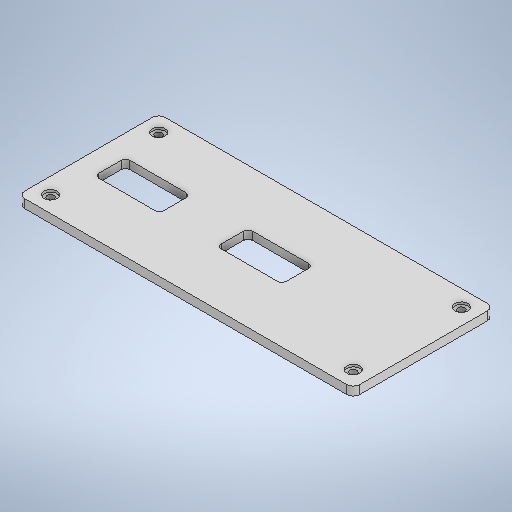
# Autodesk Inventor part: arcade_box_lid_iteration3
Saved by Autodesk Inventor 2025.2 (Build 292293000, 293)
## iProperties
Created: 2025-03-25
Part Number: arcade_box_lid_iteration3
Material: Generic
Document SubType Name: Modeling
Designer: osmon
Density: 1 g/cm^3
Appearance: Default
Author: osmon
Autodesk Inventor part; units mm, degrees
ref_plane "YZ Plane" through (0, 0, 0) normal (1, 0, 0) x (0, 1, 0)
ref_plane "XZ Plane" through (0, 0, 0) normal (0, 1, 0) x (-1, 0, 0)
ref_plane "XY Plane" through (0, 0, 0) normal (0, 0, 1) x (1, 0, 0)
sketch "Sketch1" plane through (0, 0, 0) normal (0, 1, 0) x (-1, 0, 0)
  line L0 (0, 0) -> (-155, 0)
  line L1 (-155, 0) -> (-155, -65)
  line L2 (-155, -65) -> (0, -65)
  line L3 (0, -65) -> (0, 0)
  dimension "d0" = 155
  dimension "d1" = 65
  constraints: 8 end point, 2 parallel, 1 horizontal, 1 perpendicular
  measures "d0" distance of L2.end L1.end
  measures "d1" distance of L1.end L0.end
extrude "Extrusion1" add sketch "Sketch1" along normal blind 4
sketch "Sketch2" plane through (0, 0, 0) normal (0, -1, 0) x (1, 0, 0)
  line L0 (155, 0) -> (155, -65) projected
  line L1 (0, 0) -> (155, 0) projected
  line L2 (0, -65) -> (0, 0) projected
  line L3 (155, -65) -> (0, -65) projected
  line L4 (3, -62) -> (3, -3)
  line L5 (3, -3) -> (152, -3)
  line L6 (152, -3) -> (152, -62)
  line L7 (152, -62) -> (3, -62)
  line L8 (152, -62) -> (143, -62)
  line L9 (143, -62) -> (143, -53)
  line L10 (143, -53) -> (152, -53)
  line L11 (152, -53) -> (152, -62)
  circle A0 centre (147.5, -57.5) radius 1.6
  dimension "d4" = 3
  dimension "d5" = 9
  dimension "d6" = 9
  dimension "d7" = 3.2
  constraints: 16 end point, 2 parallel, 1 centre point, 1 horizontal, 1 perpendicular, 3 other
  measures "d4" distance between parallel lines of L3 L7
  measures "d5" distance of L9.end L10.end
  measures "d6" distance of L8.end L9.end
  measures "d7" diameter of A0
extrude "Extrusion2" cut sketch "Sketch2" against normal blind 4 contours A0
sketch "Sketch3" plane through (0, 4, 0) normal (0, 1, 0) x (1, 0, 0)
  circle A0 centre (147.5, 57.5) radius 1.6 projected
  line L0 (155, 0) -> (155, 65) projected
  line L1 (155, 65) -> (0, 65) projected
  line L2 (0, 65) -> (0, 0) projected
  line L3 (0, 0) -> (155, 0) projected
  circle A1 centre (147.5, 57.5) radius 3
  dimension "d10" = 6
  constraints: 1 centre point, 1 coincident
  measures "d10" diameter of A1
extrude "Extrusion3" cut sketch "Sketch3" against normal blind 1 contours A1
sketch "Sketch4" plane through (0, 0, 0) normal (0, -1, 0) x (1, 0, 0)
  circle A0 centre (147.5, -57.5) radius 1.6 projected
  line L0 (155, 0) -> (155, -65) projected
  line L1 (0, 0) -> (155, 0) projected
  line L2 (0, -65) -> (0, 0) projected
  line L3 (155, -65) -> (0, -65) projected
  line L4 (3, -62) -> (3, -3)
  line L5 (3, -3) -> (152, -3)
  line L6 (152, -3) -> (152, -62)
  line L7 (152, -62) -> (3, -62)
  line L8 (152, -3) -> (143, -3)
  line L9 (143, -3) -> (143, -12)
  line L10 (143, -12) -> (152, -12)
  line L11 (152, -12) -> (152, -3)
  line L12 (3, -3) -> (12, -3)
  line L13 (12, -3) -> (12, -12)
  line L14 (12, -12) -> (3, -12)
  line L15 (3, -12) -> (3, -3)
  line L16 (3, -62) -> (12, -62)
  line L17 (12, -62) -> (12, -53)
  line L18 (12, -53) -> (3, -53)
  line L19 (3, -53) -> (3, -62)
  circle A1 centre (147.5, -7.5) radius 1.6
  circle A2 centre (7.5, -7.5) radius 1.6
  circle A3 centre (7.5, -57.5) radius 1.6
  dimension "d13" = 3
  dimension "d14" = 9
  dimension "d15" = 9
  dimension "d16" = 9
  dimension "d17" = 9
  dimension "d18" = 9
  dimension "d19" = 9
  dimension "d20" = 3.2
  dimension "d21" = 3.2
  dimension "d22" = 3.2
  constraints: 32 end point, 6 parallel, 3 centre point, 3 horizontal, 3 perpendicular, 3 other
  measures "d13" distance between parallel lines of L3 L7
  measures "d14" distance of L10.end L9.end
  measures "d15" distance of L9.end L8.end
  measures "d16" distance of L13.end L14.end
  measures "d17" distance of L12.end L13.end
  measures "d18" distance of L18.end L17.end
  measures "d19" distance of L17.end L16.end
  measures "d20" diameter of A1
  measures "d21" diameter of A2
  measures "d22" diameter of A3
extrude "Extrusion4" cut sketch "Sketch4" against normal blind 4 contours A1 | A2 | A3
sketch "Sketch5" plane through (0, 4, 0) normal (0, 1, 0) x (1, 0, 0)
  circle A0 centre (7.5, 57.5) radius 1.6 projected
  circle A1 centre (7.5, 7.5) radius 1.6 projected
  circle A2 centre (147.5, 7.5) radius 1.6 projected
  circle A3 centre (147.5, 57.5) radius 3 projected
  line L0 (155, 0) -> (155, 65) projected
  line L1 (155, 65) -> (0, 65) projected
  line L2 (0, 65) -> (0, 0) projected
  line L3 (0, 0) -> (155, 0) projected
  circle A4 centre (7.5, 57.5) radius 3
  circle A5 centre (7.5, 7.5) radius 3
  circle A6 centre (147.5, 7.5) radius 3
  dimension "d25" = 6
  dimension "d26" = 6
  dimension "d27" = 6
  constraints: 3 centre point, 3 coincident
  measures "d25" diameter of A4
  measures "d26" diameter of A5
  measures "d27" diameter of A6
extrude "Extrusion5" cut sketch "Sketch5" against normal blind 1 contours A4 | A5 | A6
fillet "Fillet1" radius 3 4 edges at (0, 2, 0) (0, 2, -65) (155, 2, 0) (155, 2, -65)
sketch "Sketch6" plane through (0, 4, 0) normal (0, 1, 0) x (1, 0, 0)
  line L0 (10, 25.325) -> (40, 25.325)
  line L1 (40, 25.325) -> (40, 39.675)
  line L2 (40, 39.675) -> (10, 39.675)
  line L3 (10, 39.675) -> (10, 25.325)
  line L4 (66.65, 25.325) -> (96.65, 25.325)
  line L5 (96.65, 25.325) -> (96.65, 39.675)
  line L6 (96.65, 39.675) -> (66.65, 39.675)
  line L7 (66.65, 39.675) -> (66.65, 25.325)
  point P0 (0, 0)
  dimension "d31" = 30
  dimension "d32" = 14.35
  dimension "d33" = 30
  dimension "d34" = 14.35
  constraints: 16 end point, 4 parallel, 2 horizontal, 2 perpendicular
  measures "d31" distance of L2.end L1.end
  measures "d32" distance of L1.end L0.end
  measures "d33" distance of L6.end L5.end
  measures "d34" distance of L5.end L4.end
extrude "Extrusion6" cut sketch "Sketch6" against normal blind 4
fillet "Fillet2" radius 2 8 edges at (10, 2, -39.675) (40, 2, -39.675) (10, 2, -25.325) (40, 2, -25.325) (66.65, 2, -39.675) (96.65, 2, -39.675) (66.65, 2, -25.325) (96.65, 2, -25.325)
chamfer "Chamfer1" distance 0.3 angle 45 20 edges at (5.9, 0, -7.5) (10, 0, -32.5) (10.5858, 0, -25.9108) (25, 0, -25.325) (39.4142, 0, -25.9108) (40, 0, -32.5) (39.4142, 0, -39.0892) (25, 0, -39.675) (10.5858, 0, -39.0892) (67.2358, 0, -39.0892) (81.65, 0, -39.675) (96.0642, 0, -39.0892) (96.65, 0, -32.5) (96.0642, 0, -25.9108) (81.65, 0, -25.325) (67.2358, 0, -25.9108) (66.65, 0, -32.5) (5.9, 0, -57.5) (145.9, 0, -7.5) (145.9, 0, -57.5)
body "Solid1"
